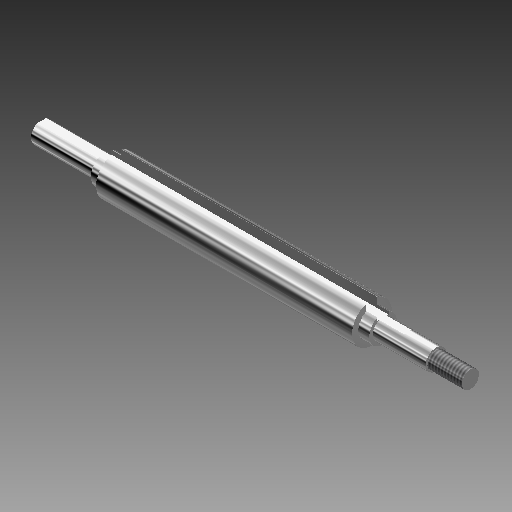
# Autodesk Inventor part: 401-01
Saved by Autodesk Inventor 2019 (Build 230136000, 136)
## iProperties
Company: Autodesk Inc.
Created: 2017-06-27
Part Number: 401-01
Material: Aluminum-6061
Document SubType Name: Modeling
Designer: Autodesk Inc.
Mass: 2.88514 g
Surface Area: 11.0585 cm^2
Volume: 1.06857 cm^3
Density: 2.7 g/cm^3
Appearance: Chrome - Polished
Author: Inventor
Autodesk Inventor part; units mm, degrees
ref_plane "YZ Plane" through (0, 0, 0) normal (1, 0, 0) x (0, 1, 0)
ref_plane "XZ Plane" through (0, 0, 0) normal (0, 1, 0) x (-1, 0, 0)
ref_plane "XY Plane" through (0, 0, 0) normal (0, 0, 1) x (1, 0, 0)
sketch "Sketch1" plane through (0, 0, 0) normal (0, 0, 1) x (1, 0, 0)
  line L0 (-18.6, 0) -> (18.6, 0)
  line L1 (18.6, 0) -> (18.6, 2.9)
  line L2 (18.6, 2.9) -> (-18.6, 2.9)
  line L3 (-18.6, 2.9) -> (-18.6, 0)
  line L4 (-18.6, 0) -> (-20.1, 0)
  line L5 (-20.1, 0) -> (-20.1, 2.15)
  line L6 (-20.1, 2.15) -> (-18.6, 2.15)
  line L7 (-18.6, 2.15) -> (-18.6, 0)
  line L8 (-20.1, 0) -> (-29.4, 0)
  line L9 (-29.4, 0) -> (-29.4, 1.55)
  line L10 (-29.4, 1.55) -> (-20.1, 1.55)
  line L11 (-20.1, 1.55) -> (-20.1, 0)
  line L12 (18.6, 0) -> (20.2, 0)
  line L13 (20.2, 0) -> (20.2, 2)
  line L14 (20.2, 2) -> (18.6, 2)
  line L15 (18.6, 2) -> (18.6, 0)
  line L16 (20.2, 0) -> (27.9, 0)
  line L17 (27.9, 0) -> (27.9, 1.5)
  line L18 (27.9, 1.5) -> (20.2, 1.5)
  line L19 (20.2, 1.5) -> (20.2, 0)
  line L20 (27.9, 0) -> (32.9, 0)
  line L21 (32.9, 0) -> (32.9, 1.25)
  line L22 (32.9, 1.25) -> (27.9, 1.25)
  line L23 (27.9, 1.25) -> (27.9, 0)
  point P0 (0, 0)
  point P1 (0, 0)
  dimension "d0" = 9.3
  dimension "d1" = 10.8
  dimension "d2" = 48
  dimension "d3" = 3.1
  dimension "d4" = 4.3
  dimension "d5" = 5.8
  dimension "d6" = 3
  dimension "d7" = 49.6
  dimension "d26" = 2.5
  dimension "d27" = 5
  dimension "d28" = 62.3
  dimension "d29" = 4
  constraints: 48 end point, 12 parallel, 6 horizontal, 6 perpendicular, 1 coincident, 1 midpoint
  measures "d0" distance of L9.end L10.end
  measures "d1" distance between parallel lines of L3 L9
  measures "d2" distance between parallel lines of L1 L9
  measures "d3" diameter of L10 L8
  measures "d4" diameter of L6 L8
  measures "d5" diameter of L2 L8
  measures "d6" diameter of L18 L16
  measures "d7" distance between parallel lines of L19 L9
  measures "d26" diameter of L22 L20
  measures "d27" distance of L21.end L22.end
  measures "d28" distance from line of L20.end L9
  measures "d29" diameter of L14 L12
revolve "Revolution1" add sketch "Sketch1" angle 360 about axis through (-18.6, 0, 0) along (1, 0, 0)
thread "Thread1" size "M2.5x0.45" class "6g" standard "ANSI Metric M Profile" length 5
hole "Hole1" at (-29.4, 0, 0) direction (1, 0, 0) diameter 1.567 depth 6 tip angle 118 counterbore diameter 1.9 counterbore depth 2 thread size "M2x0.4" class "6H" standard "ANSI Metric M Profile"
sketch "Sketch2" plane through (-29.4, 0, 0) normal (-1, 0, 0) x (0, 0, 1)
  circle A0 centre (0, 0) radius 2.9 projected
  line L0 (-0.8, 2.7875) -> (0.8, 2.7875)
  line L1 (0.8, 2.7875) -> (0.8, 1.4)
  line L2 (0.8, 1.4) -> (-0.8, 1.4)
  line L3 (-0.8, 1.4) -> (-0.8, 2.7875)
  dimension "d22" = 1.6
  dimension "d25" = 4.3
  constraints: 8 end point, 2 parallel, 2 point on circle, 1 horizontal, 1 perpendicular
  measures "d22" distance of L0.start L0.end
extrude "Extrusion1" cut sketch "Sketch2" against normal blind 53.23 contours L0 A0 | L1 L2 L3 L0
body "Solid1"
